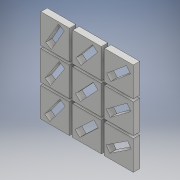
# Autodesk Inventor part: magnet-54-offset-36
Saved by Autodesk Inventor 2018 (Build 220112000, 112)
## iProperties
Created: 2025-03-17
Part Number: magnet-54-offset-36
Material: Generic
Document SubType Name: Modeling
Designer: neo
Density: 1 g/cm^3
Appearance: Default
Author: neo
Autodesk Inventor part; units mm, degrees
ref_plane "YZ Plane" through (0, 0, 0) normal (1, 0, 0) x (0, 1, 0)
ref_plane "XZ Plane" through (0, 0, 0) normal (0, 1, 0) x (-1, 0, 0)
ref_plane "XY Plane" through (0, 0, 0) normal (0, 0, 1) x (1, 0, 0)
sketch "Sketch1" plane through (0, 0, 0) normal (0, 1, 0) x (-1, 0, 0)
  line L0 (44.286, 57.5056) -> (-1.714, 57.5056)
  line L1 (-1.714, 57.5056) -> (-1.714, 11.5056)
  line L2 (-1.714, 11.5056) -> (44.286, 11.5056)
  line L3 (44.286, 11.5056) -> (44.286, 57.5056)
  line L4 (21.286, 57.5056) -> (21.286, 11.5056) construction
  line L5 (44.286, 34.5056) -> (-1.714, 34.5056) construction
  line L6 (4.8713, 45.3017) -> (21.286, 34.5056) construction
  line L7 (21.286, 34.5056) -> (15.7062, 26.0218) construction
  line L8 (7.2809, 49.8809) -> (1.6209, 41.2754)
  line L9 (1.6209, 41.2754) -> (35.2911, 19.1302)
  line L10 (35.2911, 19.1302) -> (40.951, 27.7357)
  line L11 (40.951, 27.7357) -> (7.2809, 49.8809)
  line L12 (94.286, 57.5056) -> (48.286, 57.5056)
  line L13 (48.286, 57.5056) -> (48.286, 11.5056)
  line L14 (48.286, 11.5056) -> (94.286, 11.5056)
  line L15 (94.286, 11.5056) -> (94.286, 57.5056)
  line L16 (71.286, 57.5056) -> (71.286, 11.5056) construction
  line L17 (94.286, 34.5056) -> (48.286, 34.5056) construction
  line L18 (56.9954, 47.988) -> (71.286, 34.5056) construction
  line L19 (71.286, 34.5056) -> (64.3177, 27.1196) construction
  line L20 (60.1636, 52.0793) -> (53.0953, 44.5874)
  line L21 (53.0953, 44.5874) -> (82.4084, 16.9318)
  line L22 (82.4084, 16.9318) -> (89.4767, 24.4238)
  line L23 (89.4767, 24.4238) -> (60.1636, 52.0793)
  line L24 (144.286, 57.5056) -> (98.286, 57.5056)
  line L25 (98.286, 57.5056) -> (98.286, 11.5056)
  line L26 (98.286, 11.5056) -> (144.286, 11.5056)
  line L27 (144.286, 11.5056) -> (144.286, 57.5056)
  line L28 (121.286, 57.5056) -> (121.286, 11.5056) construction
  line L29 (144.286, 34.5056) -> (98.286, 34.5056) construction
  line L30 (109.5537, 50.2647) -> (121.286, 34.5056) construction
  line L31 (121.286, 34.5056) -> (113.141, 28.4419) construction
  line L32 (113.3842, 53.7437) -> (105.1223, 47.593)
  line L33 (105.1223, 47.593) -> (129.1878, 15.2674)
  line L34 (129.1878, 15.2674) -> (137.4497, 21.4182)
  line L35 (137.4497, 21.4182) -> (113.3842, 53.7437)
  line L36 (44.286, 107.5056) -> (-1.714, 107.5056)
  line L37 (-1.714, 107.5056) -> (-1.714, 61.5056)
  line L38 (-1.714, 61.5056) -> (44.286, 61.5056)
  line L39 (44.286, 61.5056) -> (44.286, 107.5056)
  line L40 (21.286, 107.5056) -> (21.286, 61.5056) construction
  line L41 (44.286, 84.5056) -> (-1.714, 84.5056) construction
  line L42 (5.5268, 96.2378) -> (21.286, 84.5056) construction
  line L43 (21.286, 84.5056) -> (15.2223, 76.3606) construction
  line L44 (8.1986, 100.6693) -> (2.0478, 92.4074)
  line L45 (2.0478, 92.4074) -> (34.3734, 68.3419)
  line L46 (34.3734, 68.3419) -> (40.5241, 76.6038)
  line L47 (40.5241, 76.6038) -> (8.1986, 100.6693)
  line L48 (44.286, 157.5056) -> (-1.714, 157.5056)
  line L49 (-1.714, 157.5056) -> (-1.714, 111.5056)
  line L50 (-1.714, 111.5056) -> (44.286, 111.5056)
  line L51 (44.286, 111.5056) -> (44.286, 157.5056)
  line L52 (21.286, 157.5056) -> (21.286, 111.5056) construction
  line L53 (44.286, 134.5056) -> (-1.714, 134.5056) construction
  line L54 (6.2357, 147.1343) -> (21.286, 134.5056) construction
  line L55 (21.286, 134.5056) -> (14.759, 126.727) construction
  line L56 (9.1606, 151.4029) -> (2.5398, 143.5126)
  line L57 (2.5398, 143.5126) -> (33.4114, 117.6083)
  line L58 (33.4114, 117.6083) -> (40.0321, 125.4985)
  line L59 (40.0321, 125.4985) -> (9.1606, 151.4029)
  line L60 (94.286, 107.5056) -> (48.286, 107.5056)
  line L61 (48.286, 107.5056) -> (48.286, 61.5056)
  line L62 (48.286, 61.5056) -> (94.286, 61.5056)
  line L63 (94.286, 61.5056) -> (94.286, 107.5056)
  line L64 (71.286, 107.5056) -> (71.286, 61.5056) construction
  line L65 (94.286, 84.5056) -> (48.286, 84.5056) construction
  line L66 (57.8035, 98.7961) -> (71.286, 84.5056) construction
  line L67 (71.286, 84.5056) -> (63.9001, 77.5373) construction
  line L68 (61.2042, 102.6963) -> (53.7123, 95.628)
  line L69 (53.7123, 95.628) -> (81.3678, 66.3148)
  line L70 (81.3678, 66.3148) -> (88.8597, 73.3831)
  line L71 (88.8597, 73.3831) -> (61.2042, 102.6963)
  line L72 (94.286, 157.5056) -> (48.286, 157.5056)
  line L73 (48.286, 157.5056) -> (48.286, 111.5056)
  line L74 (48.286, 111.5056) -> (94.286, 111.5056)
  line L75 (94.286, 111.5056) -> (94.286, 157.5056)
  line L76 (71.286, 157.5056) -> (71.286, 111.5056) construction
  line L77 (94.286, 134.5056) -> (48.286, 134.5056) construction
  line L78 (58.6573, 149.5559) -> (71.286, 134.5056) construction
  line L79 (71.286, 134.5056) -> (63.5074, 127.9786) construction
  line L80 (62.279, 153.2517) -> (54.3887, 146.631)
  line L81 (54.3887, 146.631) -> (80.293, 115.7594)
  line L82 (80.293, 115.7594) -> (88.1833, 122.3801)
  line L83 (88.1833, 122.3801) -> (62.279, 153.2517)
  line L84 (144.286, 107.5056) -> (98.286, 107.5056)
  line L85 (98.286, 107.5056) -> (98.286, 61.5056)
  line L86 (98.286, 61.5056) -> (144.286, 61.5056)
  line L87 (144.286, 61.5056) -> (144.286, 107.5056)
  line L88 (121.286, 107.5056) -> (121.286, 61.5056) construction
  line L89 (144.286, 84.5056) -> (98.286, 84.5056) construction
  line L90 (110.4899, 100.9202) -> (121.286, 84.5056) construction
  line L91 (121.286, 84.5056) -> (112.8023, 78.9257) construction
  line L92 (114.5162, 104.1706) -> (105.9106, 98.5107)
  line L93 (105.9106, 98.5107) -> (128.0558, 64.8405)
  line L94 (128.0558, 64.8405) -> (136.6614, 70.5005)
  line L95 (136.6614, 70.5005) -> (114.5162, 104.1706)
  line L96 (144.286, 157.5056) -> (98.286, 157.5056)
  line L97 (98.286, 157.5056) -> (98.286, 111.5056)
  line L98 (98.286, 111.5056) -> (144.286, 111.5056)
  line L99 (144.286, 111.5056) -> (144.286, 157.5056)
  line L100 (121.286, 157.5056) -> (121.286, 111.5056) construction
  line L101 (144.286, 134.5056) -> (98.286, 134.5056) construction
  line L102 (111.4626, 151.5202) -> (121.286, 134.5056) construction
  line L103 (121.286, 134.5056) -> (112.4922, 129.4285) construction
  line L104 (115.671, 154.531) -> (106.751, 149.381)
  line L105 (106.751, 149.381) -> (126.901, 114.4802)
  line L106 (126.901, 114.4802) -> (135.821, 119.6302)
  line L107 (135.821, 119.6302) -> (115.671, 154.531)
  dimension "w" = 46
  dimension "d65" = 46
  dimension "d" = 10.3
  dimension "d67" = 40.3
  dimension "d68" = 146.667
  dimension "d69" = 46
  dimension "d70" = 46
  dimension "d71" = 10.3
  dimension "d72" = 40.3
  dimension "d73" = 136.667
  dimension "d76" = 46
  dimension "d77" = 46
  dimension "d78" = 10.3
  dimension "d79" = 40.3
  dimension "d80" = 126.667
  dimension "d83" = 46
  dimension "d84" = 46
  dimension "d85" = 10.3
  dimension "d86" = 40.3
  dimension "d87" = 143.333
  dimension "d90" = 46
  dimension "d91" = 46
  dimension "d92" = 10.3
  dimension "d93" = 40.3
  dimension "d94" = 140
  dimension "d97" = 46
  dimension "d98" = 46
  dimension "d99" = 10.3
  dimension "d100" = 40.3
  dimension "d101" = 133.333
  dimension "d104" = 46
  dimension "d105" = 46
  dimension "d106" = 10.3
  dimension "d107" = 40.3
  dimension "d108" = 130
  dimension "d111" = 46
  dimension "d112" = 46
  dimension "d113" = 10.3
  dimension "d114" = 40.3
  dimension "d115" = 123.333
  dimension "d118" = 46
  dimension "d119" = 46
  dimension "d120" = 10.3
  dimension "d121" = 40.3
  dimension "d122" = 120
  constraints: 216 end point, 45 midpoint, 36 perpendicular, 18 equal length, 18 parallel, 9 horizontal, 18 other
  measures "w" distance of L2.end L0.start
  measures "d65" distance of L0.start L0.end
  measures "d" distance between parallel lines of L9 L11
  measures "d67" distance between parallel lines of L10 L8
  measures "d68" angle of L5 L6
  measures "d69" distance of L14.end L12.start
  measures "d70" distance of L12.start L12.end
  measures "d71" distance between parallel lines of L21 L23
  measures "d72" distance between parallel lines of L22 L20
  measures "d73" angle of L17 L18
  measures "d76" distance of L26.end L24.start
  measures "d77" distance of L24.start L24.end
  measures "d78" distance between parallel lines of L33 L35
  measures "d79" distance between parallel lines of L34 L32
  measures "d80" angle of L29 L30
  measures "d83" distance of L38.end L36.start
  measures "d84" distance of L36.start L36.end
  measures "d85" distance between parallel lines of L45 L47
  measures "d86" distance between parallel lines of L46 L44
  measures "d87" angle of L41 L42
  measures "d90" distance of L50.end L48.start
  measures "d91" distance of L48.start L48.end
  measures "d92" distance between parallel lines of L57 L59
  measures "d93" distance between parallel lines of L58 L56
  measures "d94" angle of L53 L54
  measures "d97" distance of L62.end L60.start
  measures "d98" distance of L60.start L60.end
  measures "d99" distance between parallel lines of L69 L71
  measures "d100" distance between parallel lines of L70 L68
  measures "d101" angle of L65 L66
  measures "d104" distance of L74.end L72.start
  measures "d105" distance of L72.start L72.end
  measures "d106" distance between parallel lines of L81 L83
  measures "d107" distance between parallel lines of L82 L80
  measures "d108" angle of L77 L78
  measures "d111" distance of L86.end L84.start
  measures "d112" distance of L84.start L84.end
  measures "d113" distance between parallel lines of L93 L95
  measures "d114" distance between parallel lines of L94 L92
  measures "d115" angle of L89 L90
  measures "d118" distance of L98.end L96.start
  measures "d119" distance of L96.start L96.end
  measures "d120" distance between parallel lines of L105 L107
  measures "d121" distance between parallel lines of L106 L104
  measures "d122" angle of L101 L102
extrude "Extrusion1" add sketch "Sketch1" along normal blind 10
chamfer "Chamfer1" distance 1 angle 45 18 edges at (-144.286, 10, 134.5056) (-144.286, 10, 84.5056) (-144.286, 10, 34.5056) (-94.286, 10, 134.5056) (-94.286, 10, 84.5056) (-94.286, 10, 34.5056) (-44.286, 10, 34.5056) (-44.286, 10, 84.5056) (-44.286, 10, 134.5056) (-144.286, 5, 157.5056) (-144.286, 5, 107.5056) (-144.286, 5, 57.5056) (-94.286, 5, 157.5056) (-94.286, 5, 107.5056) (-94.286, 5, 57.5056) (-44.286, 5, 157.5056) (-44.286, 5, 107.5056) (-44.286, 5, 57.5056)
equation "\"d68\" = a0 + 8 * ad"
equation "\"d73\" = a0 + 5 * ad"
equation "\"d80\" = a0 + 2 * ad"
equation "\"d87\" = a0 + 7 * ad"
equation "\"d94\" = a0 + 6 * ad"
equation "\"d101\" = a0 + 4 * ad"
equation "\"d108\" = a0 + 3 * ad"
equation "\"d115\" = a0 + ad"
equation "\"d122\" = a0 + 0 * ad"
equation "\"ad\" = 3.33333deg"
equation "\"d74\" = 0 * d75"
equation "\"d75\" = 3.333333deg"
equation "\"d81\" = 0 * d82"
equation "\"d82\" = 3.333333deg"
equation "\"d88\" = 0 * d89"
equation "\"d89\" = 3.333333deg"
equation "\"d95\" = 0 * d96"
equation "\"d96\" = 3.333333deg"
equation "\"d102\" = 0 * d103"
equation "\"d103\" = 3.333333deg"
equation "\"d109\" = 0 * d110"
equation "\"d110\" = 3.333333deg"
equation "\"d116\" = 0 * d117"
equation "\"d117\" = 3.333333deg"
equation "\"d123\" = 0 * d124"
equation "\"d124\" = 3.333333deg"
equation "\"a0\" = 120deg"
body "Solid1"
